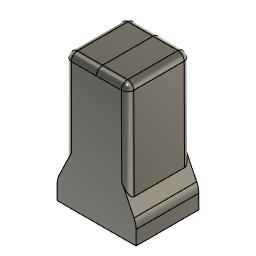
primary_007mm_select_4x (Autodesk Fusion 360 design; units mm, degrees)
Autodesk Fusion 360 part; units mm, degrees
other "Base Mesh Feature1"
sketch "Sketch1" plane through (0, 0, 0) normal (0, 0, 1) x (1, 0, 0)
other "Modify1"
sketch "Sketch2" plane through (0, 0, 0) normal (0, 1, 0) x (1, 0, 0)
  line L0 (-0.0302, -16.2862) -> (-3.8316, -16.2862)
  line L1 (-3.8316, -16.2862) -> (-3.8316, -4.3286)
  line L2 (0, -0.0002) -> (-4.8088, -0.0002)
  line L3 (-4.8088, -0.0002) -> (-4.8088, -2.3079)
  line L4 (-3.8316, -4.3286) -> (-4.8088, -2.3079)
  line L5 (0, 0) -> (0, -0.0002)
  line L6 (-0.0302, -16.2862) -> (3.7711, -16.3003)
  line L7 (3.7711, -16.3003) -> (3.8155, -4.3428)
  line L8 (3.8155, -4.3428) -> (4.8002, -2.3258)
  line L9 (4.8088, -0.018) -> (4.8002, -2.3258)
  line L10 (0, -0.0002) -> (4.8088, -0.018)
  line L11 (0, 0) -> (0, -0.0002)
  constraint horizontal L0
  constraint vertical L1
  constraint horizontal L2
  constraint vertical L3
  constraint coincident L5.start L11.start
  constraint symmetric L1.end L5 L7.end
  constraint symmetric L0.end L5 L6.end
  constraint symmetric L3.end L5 L8.end
  constraint symmetric L2.end L5 L9.start
  constraint symmetric L11.start L5 origin
  constraint symmetric L0.start L5 L6.start
extrude "Extrude1" add sketch "Sketch2" along normal mid plane 7.64 makes body 1
fillet "Fillet1" radius 0.75 10 edges at (-3.8316, 3.82, 10.3074) (-3.8316, -3.82, 10.3074) (3.7933, -3.82, 10.3215) (3.7933, 3.82, 10.3215) (3.7711, 0, 16.3003) (1.8705, -3.82, 16.2933) (-1.9309, -3.82, 16.2862) (-3.8316, 0, 16.2862) (-1.9309, 3.82, 16.2862) (1.8705, 3.82, 16.2933) on bodies 1
fillet "Fillet2" radius 2.5 2 edges at (4.8002, 0, 2.3258) (-4.8088, 0, 2.3079) on bodies 1
copy_body "Body->Comp1" bodies 1 removing the originals makes body 2 in component "primary_007mm_select_4x"
component "primary_007mm_select_4x" placed x (1, 0, 0) y (0, 1, 0) z (0, 0, 1) at (0, 0, 0)
named bodies: "primary_007mm_select_4x (1)"
